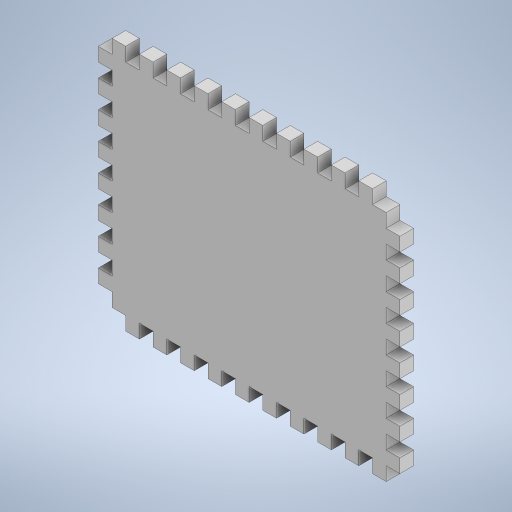
# Autodesk Inventor part: bottomside
Saved by Autodesk Inventor 2024 (Build 280153000, 153)
## iProperties
Created: 2024-04-15
Part Number: bottomside
Material: Generic
Document SubType Name: Modeling
Designer: srika
Density: 1 g/cm^3
Appearance: Default
Author: srika
Autodesk Inventor part; units mm, degrees
ref_plane "YZ Plane" through (0, 0, 0) normal (1, 0, 0) x (0, 1, 0)
ref_plane "XZ Plane" through (0, 0, 0) normal (0, 1, 0) x (-1, 0, 0)
ref_plane "XY Plane" through (0, 0, 0) normal (0, 0, 1) x (1, 0, 0)
sketch "Sketch1" plane through (0, 0, 0) normal (0, 0, 1) x (1, 0, 0)
  line L0 (5, 5) -> (105, 5)
  line L1 (105, 5) -> (105, 85)
  line L2 (105, 85) -> (5, 85)
  line L3 (5, 85) -> (5, 5)
  line L4 (0, 5) -> (5, 5)
  line L5 (5, 5) -> (5, 0)
  line L6 (5, 0) -> (0, 0)
  line L7 (0, 0) -> (0, 5)
  line L8 (0, 15) -> (5, 15)
  line L9 (5, 15) -> (5, 10)
  line L10 (5, 10) -> (0, 10)
  line L11 (0, 10) -> (0, 15)
  line L12 (0, 25) -> (5, 25)
  line L13 (5, 25) -> (5, 20)
  line L14 (5, 20) -> (0, 20)
  line L15 (0, 20) -> (0, 25)
  line L16 (0, 35) -> (5, 35)
  line L17 (5, 35) -> (5, 30)
  line L18 (5, 30) -> (0, 30)
  line L19 (0, 30) -> (0, 35)
  line L20 (0, 45) -> (5, 45)
  line L21 (5, 45) -> (5, 40)
  line L22 (5, 40) -> (0, 40)
  line L23 (0, 40) -> (0, 45)
  line L24 (0, 55) -> (5, 55)
  line L25 (5, 55) -> (5, 50)
  line L26 (5, 50) -> (0, 50)
  line L27 (0, 50) -> (0, 55)
  line L28 (0, 65) -> (5, 65)
  line L29 (5, 65) -> (5, 60)
  line L30 (5, 60) -> (0, 60)
  line L31 (0, 60) -> (0, 65)
  line L32 (0, 75) -> (5, 75)
  line L33 (5, 75) -> (5, 70)
  line L34 (5, 70) -> (0, 70)
  line L35 (0, 70) -> (0, 75)
  line L36 (0, 85) -> (5, 85)
  line L37 (5, 85) -> (5, 80)
  line L38 (5, 80) -> (0, 80)
  line L39 (0, 80) -> (0, 85)
  line L40 (10, 5) -> (15, 5)
  line L41 (15, 5) -> (15, 0)
  line L42 (15, 0) -> (10, 0)
  line L43 (10, 0) -> (10, 5)
  line L44 (20, 5) -> (25, 5)
  line L45 (25, 5) -> (25, 0)
  line L46 (25, 0) -> (20, 0)
  line L47 (20, 0) -> (20, 5)
  line L48 (30, 5) -> (35, 5)
  line L49 (35, 5) -> (35, 0)
  line L50 (35, 0) -> (30, 0)
  line L51 (30, 0) -> (30, 5)
  line L52 (40, 5) -> (45, 5)
  line L53 (45, 5) -> (45, 0)
  line L54 (45, 0) -> (40, 0)
  line L55 (40, 0) -> (40, 5)
  line L56 (50, 5) -> (55, 5)
  line L57 (55, 5) -> (55, 0)
  line L58 (55, 0) -> (50, 0)
  line L59 (50, 0) -> (50, 5)
  line L60 (60, 5) -> (65, 5)
  line L61 (65, 5) -> (65, 0)
  line L62 (65, 0) -> (60, 0)
  line L63 (60, 0) -> (60, 5)
  line L64 (70, 5) -> (75, 5)
  line L65 (75, 5) -> (75, 0)
  line L66 (75, 0) -> (70, 0)
  line L67 (70, 0) -> (70, 5)
  line L68 (80, 5) -> (85, 5)
  line L69 (85, 5) -> (85, 0)
  line L70 (85, 0) -> (80, 0)
  line L71 (80, 0) -> (80, 5)
  line L72 (90, 5) -> (95, 5)
  line L73 (95, 5) -> (95, 0)
  line L74 (95, 0) -> (90, 0)
  line L75 (90, 0) -> (90, 5)
  line L76 (100, 5) -> (105, 5)
  line L77 (105, 5) -> (105, 0)
  line L78 (105, 0) -> (100, 0)
  line L79 (100, 0) -> (100, 5)
  line L80 (105, 90) -> (110, 90)
  line L81 (110, 90) -> (110, 85)
  line L82 (110, 85) -> (105, 85)
  line L83 (105, 85) -> (105, 90)
  line L84 (100, 85) -> (95, 85)
  line L85 (95, 85) -> (95, 90)
  line L86 (95, 90) -> (100, 90)
  line L87 (100, 90) -> (100, 85)
  line L88 (90, 85) -> (85, 85)
  line L89 (85, 85) -> (85, 90)
  line L90 (85, 90) -> (90, 90)
  line L91 (90, 90) -> (90, 85)
  line L92 (80, 85) -> (75, 85)
  line L93 (75, 85) -> (75, 90)
  line L94 (75, 90) -> (80, 90)
  line L95 (80, 90) -> (80, 85)
  line L96 (70, 85) -> (65, 85)
  line L97 (65, 85) -> (65, 90)
  line L98 (65, 90) -> (70, 90)
  line L99 (70, 90) -> (70, 85)
  line L100 (60, 85) -> (55, 85)
  line L101 (55, 85) -> (55, 90)
  line L102 (55, 90) -> (60, 90)
  line L103 (60, 90) -> (60, 85)
  line L104 (50, 85) -> (45, 85)
  line L105 (45, 85) -> (45, 90)
  line L106 (45, 90) -> (50, 90)
  line L107 (50, 90) -> (50, 85)
  line L108 (40, 85) -> (35, 85)
  line L109 (35, 85) -> (35, 90)
  line L110 (35, 90) -> (40, 90)
  line L111 (40, 90) -> (40, 85)
  line L112 (30, 85) -> (25, 85)
  line L113 (25, 85) -> (25, 90)
  line L114 (25, 90) -> (30, 90)
  line L115 (30, 90) -> (30, 85)
  line L116 (20, 85) -> (15, 85)
  line L117 (15, 85) -> (15, 90)
  line L118 (15, 90) -> (20, 90)
  line L119 (20, 90) -> (20, 85)
  line L120 (10, 85) -> (5, 85)
  line L121 (5, 85) -> (5, 90)
  line L122 (5, 90) -> (10, 90)
  line L123 (10, 90) -> (10, 85)
  line L124 (110, 75) -> (105, 75)
  line L125 (105, 80) -> (110, 80)
  line L126 (110, 80) -> (110, 75)
  line L127 (105, 75) -> (105, 80)
  line L128 (110, 65) -> (105, 65)
  line L129 (105, 70) -> (110, 70)
  line L130 (110, 70) -> (110, 65)
  line L131 (105, 65) -> (105, 70)
  line L132 (110, 55) -> (105, 55)
  line L133 (105, 60) -> (110, 60)
  line L134 (110, 60) -> (110, 55)
  line L135 (105, 55) -> (105, 60)
  line L136 (110, 45) -> (105, 45)
  line L137 (105, 50) -> (110, 50)
  line L138 (110, 50) -> (110, 45)
  line L139 (105, 45) -> (105, 50)
  line L140 (110, 35) -> (105, 35)
  line L141 (105, 40) -> (110, 40)
  line L142 (110, 40) -> (110, 35)
  line L143 (105, 35) -> (105, 40)
  line L144 (110, 25) -> (105, 25)
  line L145 (105, 30) -> (110, 30)
  line L146 (110, 30) -> (110, 25)
  line L147 (105, 25) -> (105, 30)
  line L148 (110, 15) -> (105, 15)
  line L149 (105, 20) -> (110, 20)
  line L150 (110, 20) -> (110, 15)
  line L151 (105, 15) -> (105, 20)
  line L152 (110, 5) -> (105, 5)
  line L153 (105, 10) -> (110, 10)
  line L154 (110, 10) -> (110, 5)
  line L155 (105, 5) -> (105, 10)
  dimension "d4" = 10
  dimension "d11" = 10
  dimension "d18" = 10
  dimension "d25" = 10
  constraints: 308 end point, 100 horizontal alignment, 45 parallel, 40 collinear, 3 vertical, 2 horizontal, 2 perpendicular, 150 other
  measures "d4" distance of L3.end point (5, 15)
  measures "d11" distance of L3.end point (15, 5)
  measures "d18" distance of L1.end point (95, 85)
  measures "d25" distance of L1.end point (105, 75)
extrude "Extrusion1" add sketch "Sketch1" along normal blind 5 contours L3 L2 L1 L0 | L0 L41 L42 L43 | L10 L11 L8 L3 | L0 L45 L46 L47 | L14 L15 L12 L3 | L0 L49 L50 L51 | L18 L19 L16 L3 | L0 L53 L54 L55 | L22 L23 L20 L3 | L0 L57 L58 L59 | L26 L27 L24 L3 | L0 L61 L62 L63 | L30 L31 L28 L3 | L0 L65 L66 L67 | L34 L35 L32 L3 | L0 L69 L70 L71 | L38 L39 L36 L3 | L121 L122 L123 L2 | L0 L73 L74 L75 | L117 L118 L119 L2 | L0 L77 L78 L79 | L1 L153 L154 L152 | L113 L114 L115 L2 | L1 L149 L150 L148 | L109 L110 L111 L2 | L1 L145 L146 L144 | L105 L106 L107 L2 | L1 L141 L142 L140 | L101 L102 L103 L2 | L1 L137 L138 L136 | L97 L98 L99 L2 | L1 L133 L134 L132 | L93 L94 L95 L2 | L1 L129 L130 L128 | L89 L90 L91 L2 | L1 L125 L126 L124 | L85 L86 L87 L2
body "Solid1"
